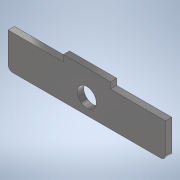
# Autodesk Inventor part: 0 零件
Saved by Autodesk Inventor 2020 (Build 240168000, 168)
## iProperties
Created: 2020-11-03
Part Number: 0 零件
Material: 不鏽鋼
Document SubType Name: Sheet Metal
Designer: p2013
Density: 8 g/cm^3
Appearance: 不鏽鋼 - 疏刷
Sheet Metal Rule: 預設 mm (_M)
Author: p2013
Autodesk Inventor part; units mm, degrees
ref_plane "YZ Plane" through (0, 0, 0) normal (1, 0, 0) x (0, 1, 0)
ref_plane "XZ Plane" through (0, 0, 0) normal (0, 1, 0) x (-1, 0, 0)
ref_plane "XY Plane" through (0, 0, 0) normal (0, 0, 1) x (1, 0, 0)
sketch "草圖1" plane through (0, 0, 0) normal (0, 0, 1) x (1, 0, 0)
  line L0 (0, 0) -> (-25.6572, 0) construction
  line L1 (0, 0) -> (0, 25.6407) construction
  line L2 (-23.5, -5.5) -> (-13.1185, -5.5)
  line L3 (25, -4) -> (25, 5.5)
  line L4 (25, 5.5) -> (-25, 5.5)
  line L5 (-25, 5.5) -> (-25, -4)
  line L6 (-25, -5.5) -> (25, 5.5) construction
  line L7 (25, -5.5) -> (-25, 5.5) construction
  arc A0 (23.5, -5.5) -> (25, -4) centre (23.5, -4) ccw
  arc A1 (-25, -4) -> (-23.5, -5.5) centre (-23.5, -4) ccw
  line L8 (-13.1185, -5.5) -> (23.5, -5.5)
  line L9 (7.5, 5.5) -> (7.5, 7.5)
  line L10 (7.5, 7.5) -> (-7.5, 7.5)
  line L11 (-7.5, 7.5) -> (-7.5, 5.5)
  circle A2 centre (0, -0.5) radius 3
  dimension "d0" = 50
  dimension "d4" = 1.5
  dimension "d13" = 2
  dimension "d14" = 15
  dimension "d15" = 6
  dimension "d16" = 6
  dimension "d17" = 5
  constraints: 24 end point, 11 point on line, 6 tangent, 4 parallel, 4 point on circle, 3 centre point, 3 horizontal, 2 midpoint, 2 perpendicular, 2 vertical, 1 equal radius, 1 other
  measures "d0" distance between parallel lines of L3 L5
  measures "d4" radius of A0
  measures "d13" distance between parallel lines of L4 L10
  measures "d14" distance between parallel lines of L11 L9
  measures "d15" diameter of A2
  measures "d16" distance from line of L4 A2.centre
  measures "d17" distance from line of A2.centre L8
extrude "擠出1" add sketch "草圖1" along normal mid plane 2
equation "\"d4\" = d5"
equation "\"折彎半徑\" = 厚度"
equation "\"折彎離隙寬度\" = 厚度"
equation "\"折彎離隙深度\" = 0.5 * 厚度"
equation "\"最小剩餘\" = 2 * 厚度"
equation "\"轉移半徑\" = 折彎半徑"
equation "\"Jacobi半徑大小\" = 折彎半徑"
equation "\"間隙大小\" = 厚度"
equation "\"d5\" = 1.5"
equation "\"厚度\" = 2.5"
